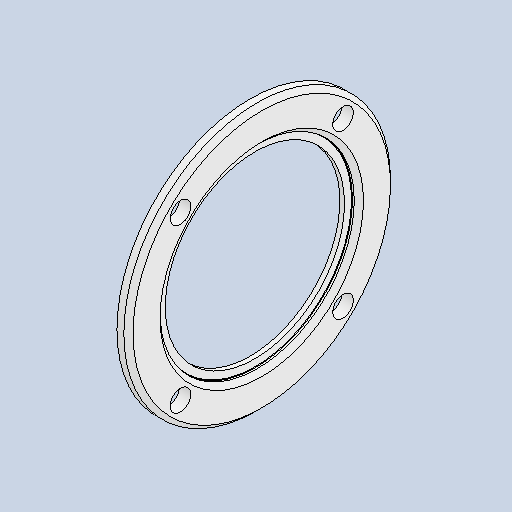
# Autodesk Inventor part: joint3_frame_cover
Saved by Autodesk Inventor 2025.3 (Build 293356030, 356C)
## iProperties
Created: 2025-11-20
Part Number: joint3_frame_cover
Material: PLA filament
Document SubType Name: Modeling
Designer: MSI
Mass: 3.58968 g
Surface Area: 34.9607 cm^2
Volume: 2.9914 cm^3
Density: 1.2 g/cm^3
Appearance: 일반
Author: MSI
Autodesk Inventor part; units mm, degrees
ref_plane "YZ Plane" through (0, 0, 0) normal (1, 0, 0) x (0, 1, 0)
ref_plane "XZ Plane" through (0, 0, 0) normal (0, 1, 0) x (-1, 0, 0)
ref_plane "XY Plane" through (0, 0, 0) normal (0, 0, 1) x (1, 0, 0)
sketch "스케치1" plane through (0, 0, 0) normal (1, 0, 0) x (0, 1, 0)
  circle A0 centre (0, 0) radius 29
  dimension "d0" = 58
  constraints: 1 centre point, 1 coincident
  measures "d0" diameter of A0
extrude "돌출1" add sketch "스케치1" along normal blind 2.5
sketch "스케치2" plane through (0, 0, 0) normal (-1, 0, 0) x (0, 0, 1)
  circle A0 centre (0, 0) radius 29 projected
  constraints: 1 coincident
hole "구멍1" at (0, 0, 0) direction (1, 0, 0) diameter 39 end through all
sketch "스케치4" plane through (2.5, 0, 0) normal (1, 0, 0) x (0, 0, -1)
  circle A0 centre (0, 0) radius 29 projected
  constraints: 1 coincident
hole "구멍3" at (2.5, 0, 0) direction (-1, 0, 0) diameter 42.25 depth 1.5
sketch "스케치3" plane through (0, 0, 0) normal (-1, 0, 0) x (0, 0, 1)
  line L0 (0, 0) -> (17.6777, 17.6777)
  line L1 (0, 0) -> (25, 0) construction
  dimension "d13" = 25
  dimension "d14" = 45
  constraints: 4 end point, 1 coincident, 1 equal length, 1 horizontal
  measures "d13" distance of L0.start L0.end
  measures "d14" angle of L1 L0
hole "구멍2" at (0, 17.6777, 17.6777) direction (1, 0, 0) diameter 4.5 end through all clearance for "Socket Head Cap Screw ISO 4762" size "M4" standard "ISO"
pattern_circular "원형 패턴1" count 4 over 360 about axis through (82.0625, 0, 0) along (-1, 0, 0) of "구멍2"
chamfer "모따기1" distance 1 angle 45 2 edges at (2.5, -29, 0) (2.5, 0, 21.125)
fillet "모깎기1" radius 0.1 1 edges at (1, 0, 21.125)
equation "\"joint4_belt_centor\" = 157.367"
equation "\"joint4_axis2_L\" = 58.803"
equation "\"joint4_axis2_b1\" = 35"
equation "\"joint4_axis2_d\" = 19"
equation "\"joint4_miter_m\" = 2"
equation "\"joint4_miter_a\" = 20deg"
equation "\"joint4_miter_z\" = 79"
equation "\"joint4_miter_b\" = 6.90139"
equation "\"joint4_axis3_L\" = 23.5"
equation "\"joint3_belt_centor\" = 157.367"
equation "\"joint3_axis2_L\" = 63.75"
equation "\"joint3_axis2_b1\" = 38"
equation "\"joint3_axis2_d\" = 29"
equation "\"joint3_planetary_m\" = 2"
equation "\"joint3_planetary_a\" = 20deg"
equation "\"joint3_planetary_np\" = 4"
equation "\"joint3_sun_b\" = 19"
equation "\"joint3_planet_b\" = 19"
equation "\"joint3_ring_b\" = 18"
equation "\"joint3_axis3_d\" = 29"
equation "\"joint3_miter_m\" = 4"
equation "\"joint3_miter_a\" = 20deg"
equation "\"joint3_miter_z1\" = 26"
equation "\"joint3_miter_z2\" = 39"
equation "\"joint3_miter_b\" = 25.07657"
equation "\"joint3_axis4_L\" = 43.706"
